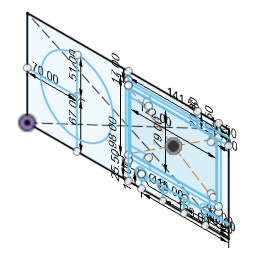
PiRetroRadio (Autodesk Fusion 360 design; units mm, degrees)
Autodesk Fusion 360 part; units mm, degrees
sketch "Base" plane through (0, 0, 0) normal (0, 1, 0) x (1, 0, 0)
  line L0 (284, 0) -> (0, 0)
  line L1 (0, 0) -> (0, -134)
  line L2 (0, -134) -> (284, -134)
  line L3 (284, -134) -> (284, 0)
  line L4 (284, 0) -> (0, -134) construction
  line L5 (0, 0) -> (284, -134) construction
  circle A0 centre (251, -18) radius 7.5
  circle A1 centre (221, -18) radius 7.5
  circle A2 centre (161, -18) radius 7.5
  circle A3 centre (191, -18) radius 7.5
  circle A4 centre (161, -18) radius 3.75
  circle A5 centre (191, -18) radius 3.75
  circle A6 centre (221, -18) radius 3.75
  circle A7 centre (251, -18) radius 3.75
  circle A8 centre (70, -67) radius 51
  dimension "d1" = 284
  dimension "d2" = 134
  dimension "d3" = 15
  dimension "d7" = 15
  dimension "d9" = 15
  dimension "d10" = 15
  dimension "d29" = -3.75
  dimension "d30" = -3.75
  dimension "d31" = -3.75
  dimension "d32" = -3.75
  dimension "d135" = 102
  constraint horizontal L0
  constraint perpendicular L0 L1
  constraint parallel L0 L2
  constraint parallel L1 L3
  constraint coincident L0.end L1.start
  measures "d1" distance of L1.end L2.end
  measures "d2" distance of L0.end L1.end
  measures "d3" diameter of A0
  measures "d7" diameter of A1
  measures "d9" diameter of A2
  measures "d10" diameter of A3
  measures "d135" diameter of A8
sketch "Front Frame" plane through (0, 0, 0) normal (0, 1, 0) x (1, 0, 0)
  line L0 (152, -110) -> (259.5, -110)
  line L1 (259.5, -110) -> (259.5, -45)
  line L2 (259.5, -45) -> (152, -45)
  line L3 (152, -45) -> (152, -110)
  line L4 (139, -127) -> (273, -127)
  line L5 (273, -127) -> (273, -7)
  line L6 (273, -7) -> (139, -7)
  line L7 (139, -7) -> (139, -127)
  dimension "d75" = 107.5
  dimension "d76" = 65
  dimension "d77" = 134
  dimension "d78" = 120
  constraint horizontal L0
  constraint vertical L1
  constraint horizontal L2
  constraint vertical L3
  constraint horizontal L4
  constraint vertical L5
  constraint horizontal L6
  constraint vertical L7
  measures "d75" distance of L0.start L0.end
  measures "d76" distance of L0.start L2.end
  measures "d77" distance of L4.start L4.end
  measures "d78" distance of L4.start L6.end
sketch "Back Frame" plane through (0, 0, 0) normal (0, 1, 0) x (1, 0, 0)
  line L0 (145, -35) -> (145, -114)
  line L1 (145, -35) -> (173, -35)
  line L2 (145, -35) -> (145, -114)
  arc A0 (173, -106) -> (171, -104) centre (171, -106) ccw
  line L3 (173, -35) -> (173, -43)
  line L4 (139, -29) -> (139, -120)
  line L5 (145, -104) -> (145, -114)
  arc A1 (171, -45) -> (173, -43) centre (171, -43) ccw
  line L6 (171, -104) -> (145, -104)
  line L7 (267, -35) -> (145, -114) construction
  line L8 (145, -35) -> (267, -114) construction
  line L9 (139, -120) -> (273, -120)
  line L10 (267, -35) -> (145, -35)
  arc A2 (259, -104) -> (257, -106) centre (259, -106) ccw
  line L11 (257, -114) -> (257, -106)
  line L12 (257, -35) -> (257, -43)
  line L13 (171, -45) -> (145, -45)
  circle A3 centre (262, -39.8) radius 1.25
  line L14 (145, -114) -> (173, -114)
  arc A4 (257, -43) -> (259, -45) centre (259, -43) ccw
  circle A5 centre (262, -109.8) radius 1.25
  line L15 (267, -35) -> (145, -35)
  line L16 (145, -114) -> (267, -114)
  line L17 (145, -114) -> (267, -114)
  line L18 (267, -35) -> (257, -35)
  line L19 (273, -29) -> (139, -29)
  line L20 (145, -45) -> (145, -35)
  circle A6 centre (168.7, -39.8) radius 1.25
  line L21 (173, -114) -> (173, -106)
  line L22 (267, -114) -> (257, -114)
  line L23 (267, -45) -> (267, -35)
  line L24 (259, -104) -> (267, -104)
  line L25 (267, -104) -> (267, -114)
  line L26 (273, -120) -> (273, -29)
  line L27 (259, -45) -> (267, -45)
  line L28 (267, -114) -> (267, -35)
  line L29 (267, -114) -> (267, -35)
  circle A7 centre (168.7, -109.8) radius 1.25
  line L30 (139, -120) -> (146, -120)
  line L31 (146, -120) -> (146, -127)
  line L32 (146, -127) -> (139, -127)
  line L33 (139, -127) -> (139, -120)
  line L34 (273, -120) -> (266, -120)
  line L35 (266, -120) -> (266, -127)
  line L36 (266, -127) -> (273, -127)
  line L37 (273, -127) -> (273, -120)
  line L38 (139, -29) -> (146, -29)
  line L39 (146, -29) -> (146, -22)
  line L40 (146, -22) -> (139, -22)
  line L41 (139, -22) -> (139, -29)
  line L42 (273, -29) -> (266, -29)
  line L43 (266, -29) -> (266, -22)
  line L44 (266, -22) -> (273, -22)
  line L45 (273, -22) -> (273, -29)
  circle A8 centre (142.4994, -123.5) radius 1.25
  circle A9 centre (142.4994, -123.5) radius 2.75
  circle A10 centre (142.5, -25.5) radius 1.25
  circle A11 centre (142.5, -25.5) radius 2.75
  circle A12 centre (269.5, -25.5) radius 1.25
  circle A13 centre (269.5, -25.5) radius 2.75
  circle A14 centre (269.5, -123.5) radius 1.25
  circle A15 centre (269.5, -123.5) radius 2.75
  circle A16 centre (269.5, -117) radius 1.25
  circle A17 centre (269.5, -32.497) radius 1.25
  circle A18 centre (142.5, -32) radius 1.25
  circle A19 centre (142.5, -117) radius 1.25
  line L46 (257, -114) -> (257, -120)
  line L47 (257, -35) -> (257, -29)
  line L48 (173, -35) -> (173, -29)
  line L49 (173, -114) -> (173, -120)
  point P0 (206, -74.5)
  point P1 (206, -74.5)
  dimension "d82" = 79
  dimension "d83" = 2.5
  dimension "d85" = 2.5
  dimension "d86" = 2.5
  dimension "d157" = 122
  constraint horizontal L16
  constraint vertical L28
  constraint horizontal L10
  constraint vertical L0
  constraint perpendicular L2 L15
  constraint parallel L15 L17
  constraint parallel L2 L29
  constraint coincident P1 L7
  constraint coincident P1 L8
  constraint coincident P1 P0
  constraint horizontal L22
  constraint vertical L11
  constraint horizontal L24
  constraint vertical L25
  constraint horizontal L18
  constraint vertical L12
  constraint horizontal L27
  constraint vertical L23
  constraint horizontal L1
  constraint vertical L3
  constraint horizontal L13
  constraint vertical L20
  constraint horizontal L14
  constraint vertical L21
  constraint horizontal L6
  constraint vertical L5
  constraint tangent A0 L21
  constraint tangent A0 L6
  constraint tangent A2 L11
  constraint tangent A2 L24
  constraint equal A0 A2
  constraint tangent L12 A4
  constraint tangent A4 L27
  constraint equal A0 A4
  constraint tangent L3 A1
  constraint tangent A1 L13
  constraint horizontal L30
  constraint vertical L31
  constraint horizontal L32
  constraint vertical L33
  constraint horizontal L34
  constraint vertical L35
  constraint horizontal L36
  constraint vertical L37
  constraint horizontal L38
  constraint vertical L39
  constraint horizontal L40
  constraint vertical L41
  constraint horizontal L42
  constraint vertical L43
  constraint horizontal L44
  constraint vertical L45
  constraint coincident L9 L46.end
  constraint perpendicular L9 L46
  constraint coincident L19 L47.end
  constraint perpendicular L19 L47
  constraint coincident L19 L48.end
  constraint perpendicular L19 L48
  constraint coincident L9 L49.end
  constraint perpendicular L9 L49
  measures "d82" distance of L0.start L0.end
  measures "d83" diameter of A5
  measures "d85" diameter of A6
  measures "d86" diameter of A7
  measures "d157" distance of L8.end L0.end
extrude "Extrude5" add sketch "Front Frame" against normal blind 3.5 makes body 1
extrude "Extrude6" cut sketch "Base" against normal blind 4 contours A4 | A5 | A6 | A7 bodies 1
draft "Draft1" angle -20 neutral plane through (0, 0, 0) pull (0, 1, 0) 1 faces at (152, -1.1667, 66.6667) on bodies 1
draft "Draft2" angle -20 neutral plane through (0, 0, 0) pull (0, 1, 0) 1 faces at (187.4087, -2.3333, 45) on bodies 1
draft "Draft3" angle -20 neutral plane through (0, 0, 0) pull (0, 1, 0) 2 faces at (259.5, -2.3333, 66.242) (187.4087, -2.3333, 110) on bodies 1
draft "Draft4" angle -20 neutral plane through (0, 0, 0) pull (0, 1, 0) 2 faces at (273, -2.3333, 87) (183.6667, -1.1667, 127) on bodies 1
draft "Draft5" angle -20 neutral plane through (0, 0, 0) pull (0, 1, 0) 2 faces at (139, -1.1667, 86.5754) (227.9087, -1.1667, 7) on bodies 1
extrude "Extrude11" add sketch "Back Frame" along normal blind 5 and the other way blind -8.5 separate body contours L0 L1 L2 L4 L5 L9 L10 L14 L15 L16 L17 L19 L20 L30 L38 L48 L49 | L10 L15 L19 L47 L48 | L9 L10 L15 L16 L17 L18 L19 L22 L23 L25 L26 L28 L29 L34 L42 L46 L47 | L19 L38 L39 L40 L41 | L9 L16 L17 L46 L49 | L9 L30 L31 L32 L33 | L9 L34 L35 L36 L37 | A9 | A11 | A15 makes body 2
extrude "Extrude12" add sketch "Back Frame" along normal blind 7 and the other way blind -8.5 contours L0 L1 L2 L3 A1 L10 L13 L15 L20 | L0 L2 A0 L5 L6 L14 L16 L17 L21 | L10 L12 A4 L15 L18 L23 L27 L28 L29 | A2 L11 L16 L17 L22 L24 L25 L28 L29 bodies 2
sketch "Dimensions" plane through (0, 0, 0) normal (0, 1, 0) x (1, 0, 0)
  line L0 (251, -18) -> (251, 0)
  line L1 (221, -18) -> (221, 0)
  line L2 (191, -18) -> (191, 0)
  line L3 (161, -18) -> (161, 0)
  line L4 (251, -18) -> (284, -18)
  line L5 (221, -18) -> (284, -18)
  line L6 (191, -18) -> (284, -18)
  line L7 (161, -18) -> (284, -18)
  line L8 (269.5, -123.5) -> (284, -123.5)
  line L9 (269.5, -123.5) -> (269.5, -134)
  line L10 (142.5, -123.5) -> (284, -123.5)
  line L11 (142.5, -25.5) -> (142.5, 0)
  line L12 (142.5, -117) -> (142.5, -134)
  line L13 (70, -67) -> (70.5001, -118)
  line L14 (70, -67) -> (70, 0)
  line L15 (70, -67) -> (0, -67)
  line L16 (145, -114) -> (267, -114)
  line L17 (267, -114) -> (267, -35)
  line L18 (267, -35) -> (145, -35)
  line L19 (145, -35) -> (145, -114)
  line L20 (267, -114) -> (267, -35)
  line L21 (267, -114) -> (284, -114)
  line L22 (240, -114) -> (240, -134)
  line L23 (142.5, -123.5) -> (142.5, -25.5)
  circle A0 centre (161, -18) radius 7.5
  dimension "d144" = 18
  dimension "d145" = 33
  dimension "d146" = 63
  dimension "d147" = 93
  dimension "d148" = 123
  dimension "d149" = 10.5
  dimension "d150" = 14.5
  dimension "d151" = 141.5
  dimension "d152" = 25.5
  dimension "d153" = 17
  dimension "d154" = 51
  dimension "d155" = 67
  dimension "d156" = 70
  dimension "d158" = 122
  dimension "d159" = 79
  dimension "d160" = 17
  dimension "d161" = 20
  dimension "d162" = 98
  dimension "d178" = 15
  constraint vertical L0
  constraint vertical L1
  constraint vertical L2
  constraint vertical L3
  constraint perpendicular L0 L4
  constraint perpendicular L1 L5
  constraint perpendicular L1 L6
  constraint perpendicular L3 L7
  constraint horizontal L8
  constraint perpendicular L8 L9
  constraint parallel L8 L10
  constraint vertical L11
  constraint vertical L12
  constraint vertical L14
  constraint perpendicular L14 L15
  constraint horizontal L16
  constraint vertical L17
  constraint horizontal L18
  constraint vertical L19
  constraint perpendicular L17 L21
  constraint coincident L16 L22.start
  constraint perpendicular L16 L22
  constraint perpendicular L10 L23
  measures "d144" distance of L3.start L3.end
  measures "d145" distance of L0.start L4.end
  measures "d146" distance of L1.start L4.end
  measures "d147" distance of L2.start L4.end
  measures "d148" distance of L3.start L4.end
  measures "d149" distance of L8.start L9.end
  measures "d150" distance of L8.start L8.end
  measures "d151" distance of L8.end L10.start
  measures "d152" distance of L11.start L11.end
  measures "d153" distance of L12.start L12.end
  measures "d154" vertical distance of L13.start L13.end
  measures "d155" distance of L13.start L14.end
  measures "d156" distance of L13.start L15.end
  measures "d158" distance of L16.start L16.end
  measures "d159" distance of L16.start L18.end
  measures "d160" distance of L16.end L21.end
  measures "d161" distance of L22.start L22.end
  measures "d162" distance of L10.start L11.start
  measures "d178" diameter of A0
extrude "Extrude14" add sketch "Back Frame" along normal blind 8.5 and the other way blind -7 separate body contours L0 L1 L2 L3 A1 L10 L13 L15 L20 | L0 L1 L2 L4 L5 L9 L10 L14 L15 L16 L17 L19 L20 L30 L38 L48 L49 | L0 L2 A0 L5 L6 L14 L16 L17 L21 | L9 L10 L15 L16 L17 L18 L19 L22 L23 L25 L26 L28 L29 L34 L42 L46 L47 | L10 L12 A4 L15 L18 L23 L27 L28 L29 | L19 L38 L39 L40 L41 | A2 L11 L16 L17 L22 L24 L25 L28 L29 | L9 L30 L31 L32 L33 | L9 L34 L35 L36 L37 | A9 | A11 | A15 makes body 3 at (262.4167, 7, 33.349) makes body 4 at (152.823, 7, 111.339)
extrude "Extrude15" add sketch "Back Frame" along normal blind 8.5 and the other way blind -5 contours L0 L1 L2 L4 L5 L9 L10 L14 L15 L16 L17 L19 L20 L30 L38 L48 L49 | L9 L10 L15 L16 L17 L18 L19 L22 L23 L25 L26 L28 L29 L34 L42 L46 L47 | L19 L38 L39 L40 L41 | L9 L30 L31 L32 L33 | L9 L34 L35 L36 L37 | A9 | A11 | A15 bodies 3 4
extrude "Extrude16" add sketch "Back Frame" along normal blind 6 contours A9 | A11 | A15 bodies 1
extrude "Extrude7" [suppressed]
hidden bodies 1 2 3 4
named bodies: "Front Frame", "Back Frame", "Back Frame Left", "Back Frame Right"
